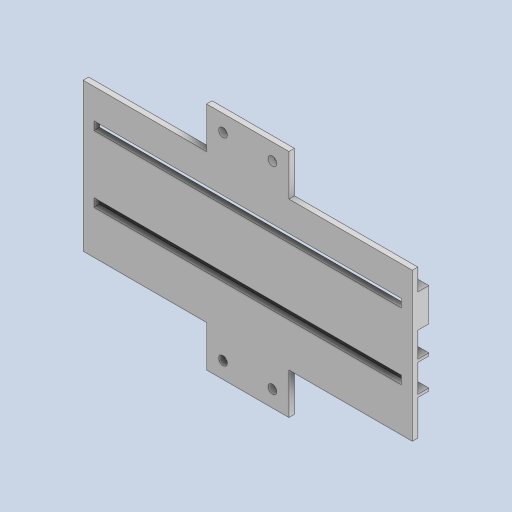
# Autodesk Inventor part: hand_box1
Saved by Autodesk Inventor 2023 (Build 270158000, 158)
## iProperties
Created: 2024-11-28
Part Number: hand_box1
Material: Generic
Document SubType Name: Modeling
Designer: kiyo
Density: 1 g/cm^3
Appearance: Default
Author: kiyo
Autodesk Inventor part; units mm, degrees
ref_plane "YZ Plane" through (0, 0, 0) normal (1, 0, 0) x (0, 1, 0)
ref_plane "XZ Plane" through (0, 0, 0) normal (0, 1, 0) x (-1, 0, 0)
ref_plane "XY Plane" through (0, 0, 0) normal (0, 0, 1) x (1, 0, 0)
sketch "スケッチ1" plane through (0, 0, 0) normal (1, 0, 0) x (0, 1, 0)
  line L0 (60, -16.042) -> (-60, -16.042)
  line L1 (-60, -16.042) -> (-60, 16.042)
  line L2 (-60, 16.042) -> (60, 16.042)
  line L3 (60, 16.042) -> (60, -16.042)
  line L4 (60, -16.042) -> (-60, 16.042) construction
  line L5 (-60, -16.042) -> (60, 16.042) construction
  line L6 (-56, 13.625) -> (56, 13.625)
  line L7 (56, 13.625) -> (56, 10.625)
  line L8 (56, 10.625) -> (-56, 10.625)
  line L9 (-56, 10.625) -> (-56, 13.625)
  line L10 (-56, -10.625) -> (56, -10.625)
  line L11 (56, -10.625) -> (56, -13.625)
  line L12 (56, -13.625) -> (-56, -13.625)
  line L13 (-56, -13.625) -> (-56, -10.625)
  line L14 (60, -16.042) -> (-60, -16.042)
  line L15 (-60, -16.042) -> (-60, -29.5)
  line L16 (-60, -29.5) -> (60, -29.5)
  line L17 (60, -29.5) -> (60, -16.042)
  line L18 (-60, 16.042) -> (60, 16.042)
  line L19 (60, 16.042) -> (60, 24.5)
  line L20 (60, 24.5) -> (-60, 24.5)
  line L21 (-60, 24.5) -> (-60, 16.042)
  line L22 (15, 24.5) -> (-15, 24.5)
  line L23 (-15, 24.5) -> (-15, 39.5)
  line L24 (-15, 39.5) -> (15, 39.5)
  line L25 (15, 39.5) -> (15, 24.5)
  line L26 (20, -29.5) -> (10, -29.5)
  line L27 (-10, -29.5) -> (-20, -29.5)
  circle A0 centre (9, 33.5) radius 1.6
  circle A1 centre (-9, 33.5) radius 1.6
  line L28 (60, 0) -> (-60, 0)
  line L29 (15, -29.5) -> (-15, -29.5)
  line L30 (-15, -29.5) -> (-15, -44.5)
  line L31 (-15, -44.5) -> (15, -44.5)
  line L32 (15, -44.5) -> (15, -29.5)
  circle A2 centre (-9, -38.5) radius 1.6
  circle A3 centre (9, -38.5) radius 1.6
  point P0 (0, 0)
  point P1 (0, 0)
  point P2 (56, 12.125)
  point P3 (56, -12.125)
  point P4 (0, 0)
  point P5 (-15, 24.5)
  point P6 (-15, -29.5)
  dimension "d1" = 120
  dimension "d3" = 12.125
  dimension "d6" = 3
  dimension "d11" = 12.125
  dimension "d15" = 2.417
  dimension "d26" = 4
  dimension "d27" = 4
  dimension "d41" = 29.5
  dimension "d53" = 54
  dimension "d72" = 15
  dimension "d74" = 15
  dimension "d75" = 30
  dimension "d79" = 6
  dimension "d80" = 3.2
  dimension "d92" = 18
  dimension "d97" = 15
  dimension "d101" = 72
  dimension "d106" = 9
  constraints: 66 end point, 14 parallel, 10 horizontal, 9 midpoint, 7 perpendicular, 5 collinear, 5 point on line, 4 centre point, 1 vertical, 6 other
  measures "d1" distance of L1.end L2.end
  measures "d3" vertical distance of point (56, -12.125) point (0, 0)
  measures "d6" distance of L8.end L6.start
  measures "d11" vertical distance of point (0, 0) point (56, 12.125)
  measures "d15" distance between parallel lines of L2 L6
  measures "d26" distance between parallel lines of L3 L7
  measures "d27" distance between parallel lines of L1 L9
  measures "d41" distance from line of L16 point (0, 0)
  measures "d53" distance between parallel lines of L16 L20
  measures "d72" distance of L22.end L23.end
  measures "d74" distance from line of point (0, 0) L23
  measures "d75" distance of L23.end L24.end
  measures "d79" distance from line of L25 A0.centre
  measures "d80" diameter of A0
  measures "d92" distance of A0.centre A1.centre
  measures "d97" distance of L29.end L30.end
  measures "d101" distance of A1.centre A2.centre
  measures "d106" distance from line of L20 A1.centre
extrude "押し出し1" add sketch "スケッチ1" along normal blind 2
sketch "スケッチ3" plane through (0, 0, 0) normal (-1, 0, 0) x (0, 0, 1)
  line L0 (-29.5, 60) -> (24.5, 60) projected
  line L1 (5.575, 60) -> (4.575, 60)
  line L2 (4.575, 60) -> (4.575, 7)
  line L3 (4.575, 7) -> (5.575, 7)
  line L4 (5.575, 7) -> (5.575, 60)
  line L5 (16.675, 60) -> (15.675, 60)
  line L6 (15.675, 60) -> (15.675, 0)
  line L7 (15.675, 0) -> (16.675, 0)
  line L8 (16.675, 0) -> (16.675, 60)
  line L9 (0, 0) -> (4.575, 0)
  line L10 (0, 0) -> (0, 19.0491)
  line L11 (5.575, -60) -> (4.575, -60)
  line L12 (4.575, -60) -> (4.575, -7)
  line L13 (4.575, -7) -> (5.575, -7)
  line L14 (5.575, -7) -> (5.575, -60)
  line L15 (16.675, -60) -> (15.675, -60)
  line L16 (15.675, -60) -> (15.675, 0)
  line L17 (16.675, 0) -> (16.675, -60)
  line L18 (-5.575, 60) -> (-4.575, 60)
  line L19 (-4.575, 60) -> (-4.575, 7)
  line L20 (-4.575, 7) -> (-5.575, 7)
  line L21 (-5.575, 7) -> (-5.575, 60)
  line L22 (-16.675, 60) -> (-15.675, 60)
  line L23 (-15.675, 60) -> (-15.675, 0)
  line L24 (-15.675, 0) -> (-16.675, 0)
  line L25 (-16.675, 0) -> (-16.675, 60)
  line L26 (-5.575, -60) -> (-4.575, -60)
  line L27 (-4.575, -60) -> (-4.575, -7)
  line L28 (-4.575, -7) -> (-5.575, -7)
  line L29 (-5.575, -7) -> (-5.575, -60)
  line L30 (-16.675, -60) -> (-15.675, -60)
  line L31 (-15.675, -60) -> (-15.675, 0)
  line L32 (-16.675, 0) -> (-16.675, -60)
  line L33 (5.575, 60) -> (15.675, 60)
  line L34 (15.675, 60) -> (15.675, 59)
  line L35 (15.675, 59) -> (5.575, 59)
  line L36 (5.575, 59) -> (5.575, 60)
  line L37 (-5.575, -60) -> (-15.675, -60)
  line L38 (-15.675, -60) -> (-15.675, -59)
  line L39 (-15.675, -59) -> (-5.575, -59)
  line L40 (-5.575, -59) -> (-5.575, -60)
  point P0 (-15.675, 60)
  point P1 (-16.675, 60)
  point P2 (15.675, 60)
  point P3 (0, 9.5245)
  point P4 (-5.575, -59)
  point P5 (5.575, 59)
  dimension "d31" = 1
  dimension "d33" = 1
  dimension "d34" = 60
  dimension "d35" = 10.1
  dimension "d36" = 7
  dimension "d61" = 5.575
  dimension "d62" = 1
  dimension "d63" = 1
  constraints: 80 end point, 20 symmetric about line, 8 parallel, 5 horizontal, 4 perpendicular, 3 point on line, 1 midpoint, 1 vertical
  measures "d31" distance of L2.end L3.end
  measures "d33" distance of L6.end L7.end
  measures "d34" distance of L7.end L5.start
  measures "d35" distance between parallel lines of L6 L4
  measures "d36" distance from line of L9.start L3
  measures "d61" distance between parallel lines of L4 L10
  measures "d62" distance between parallel lines of L0 L35
  measures "d63" distance between parallel lines of L37 L39
extrude "押し出し4" add sketch "スケッチ3" along normal blind 4
equation "\"d74\" = 0.5 * d75"
equation "\"d2\" = 0.25 * d0"
equation "\"d73\" = d72"
equation "\"d78\" = 0.5 * d72"
equation "\"d0\" = 30"
